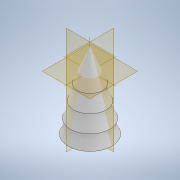
# Autodesk Inventor part: Tree_Leaves
Saved by Autodesk Inventor 2022.4 (Build 264492010, 492A)
## iProperties
Created: 2025-02-23
Part Number: Tree_Leaves
Material: Generic
Document SubType Name: Modeling
Designer: jan-m
Density: 1 g/cm^3
Appearance: Default
Author: jan-m
Autodesk Inventor part; units mm, degrees
sketch "Sketch1" plane through (0, 0, 0) normal (1, 0, 0) x (0, 1, 0)
  line L0 (20, 20) -> (-50, 20)
  line L1 (-50, 20) -> (-50, -20)
  line L2 (-50, -20) -> (20, -20)
  line L3 (20, -20) -> (20, 20)
  line L4 (-64, 0) -> (34, 0) projected
  line L5 (0, 28) -> (0, -28) projected
  line L6 (-50, 5) -> (-45, 5)
  line L7 (-45, 5) -> (-45, -5)
  line L8 (-45, -5) -> (-50, -5)
  line L9 (-50, -5) -> (-50, 5)
  line L10 (-45, 2.5) -> (-40, 2.5)
  line L11 (-40, 2.5) -> (-40, -2.5)
  line L12 (-40, -2.5) -> (-45, -2.5)
  line L13 (-45, -2.5) -> (-45, 2.5)
  line L14 (20, 0) -> (-9.519, 11.7284)
  line L15 (-9.519, 11.7284) -> (-9.519, 5)
  line L16 (20, 0) -> (-50, 0)
  line L17 (-9.519, 9.4368) -> (-23.459, 14.9754)
  line L18 (-23.459, 14.9754) -> (-23.459, 5)
  line L19 (-23.459, 12.5046) -> (-37.399, 18.0432)
  line L20 (-37.399, 18.0432) -> (-37.399, 5)
  line L21 (-37.399, 15.2739) -> (-50, 20)
  point P0 (0, 0)
  point P1 (-45, 0)
  point P2 (-40, 0)
  point P3 (0, 5)
  point P4 (0, 2.5)
  point P5 (0, 7.9463)
  dimension "d0" = 70
  dimension "d1" = 40
  dimension "d2" = 20
  dimension "d3" = 5
  dimension "d4" = 10
  dimension "d5" = 5
  dimension "d6" = 5
  dimension "d8" = 15
  dimension "d9" = 15
  constraints: 40 end point, 11 point on line, 8 parallel, 6 perpendicular, 4 midpoint, 3 horizontal
  measures "d0" distance of L2.end L1.end
  measures "d1" distance of L1.end L0.end
  measures "d2" distance between parallel lines of L5 L3
  measures "d3" distance of L7.end L8.end
  measures "d4" distance of L6.end L7.end
  measures "d5" distance of L11.end L12.end
  measures "d6" distance of L10.end L11.end
  measures "d8" distance of L17.start L17.end
  measures "d9" distance of L19.start L19.end
revolve "Revolution2" add sketch "Sketch1" angle 360 about axis through (0, 20, 0) along (0, -1, 0) contours L4 L5 L14 | L21 L20 L19 L18 L17 L15 L14 L5 L4 L11 L10 L7 L6 L1
body "Solid2"
